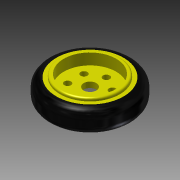
# Autodesk Inventor part: rear
Saved by Autodesk Inventor 2015 (Build 190159000, 159)
## iProperties
Created: 2015-09-11
Part Number: rear
Material: Generic
Document SubType Name: Modeling
Designer: Okorie Ifeanyichukwu
Density: 1 g/cm^3
Appearance: Smooth - Yellow
Author: Okorie Ifeanyichukwu
Autodesk Inventor part; units mm, degrees
ref_plane "YZ Plane" through (0, 0, 0) normal (1, 0, 0) x (0, 1, 0)
ref_plane "XZ Plane" through (0, 0, 0) normal (0, 1, 0) x (-1, 0, 0)
ref_plane "XY Plane" through (0, 0, 0) normal (0, 0, 1) x (1, 0, 0)
sketch "Sketch1" plane through (0, 0, 0) normal (0, 0, 1) x (1, 0, 0)
  circle A0 centre (0, 0) radius 150
  circle A1 centre (0, 0) radius 106.693
  dimension "d0" = 300
  constraints: 2 centre point, 2 coincident
  measures "d0" diameter of A0
extrude "Extrusion1" add sketch "Sketch1" along normal mid plane 80
fillet "Fillet1" radius 30 2 edges at (-150, 0, 40) (-150, 0, -40)
sketch "Sketch2" plane through (0, 0, 0) normal (0, 0, 1) x (1, 0, 0)
  circle A0 centre (0, 0) radius 106.693 projected
  circle A1 centre (0, 0) radius 93.6614
  constraints: 1 centre point, 1 coincident
extrude "Extrusion2" add sketch "Sketch2" along normal mid plane 100
fillet "Fillet2" radius 6 2 edges at (-106.693, 0, -50) (-106.693, 0, 50)
sketch "Sketch3" plane through (0, 0, 0) normal (0, 0, 1) x (1, 0, 0)
  circle A0 centre (0, 0) radius 93.6614 projected
  circle A1 centre (0, 0) radius 22.8659
  circle A2 centre (0, 58.4849) radius 11.9417
  circle A3 centre (-50.6494, 29.2425) radius 11.9417
  circle A4 centre (-50.6494, -29.2425) radius 11.9417
  circle A5 centre (0, -58.4849) radius 11.9417
  circle A6 centre (50.6494, -29.2425) radius 11.9417
  circle A7 centre (50.6494, 29.2425) radius 11.9417
  dimension "d9" = 360
  constraints: 7 centre point, 1 coincident, 13 other
extrude "Extrusion3" add sketch "Sketch3" along normal mid plane 20
body "Solid1"
